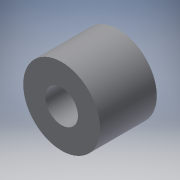
# Autodesk Inventor part: Espaçadores
Saved by Autodesk Inventor 2019 (Build 230136000, 136)
## iProperties
Created: 2020-05-30
Part Number: Espaçadores
Material: Generic
Document SubType Name: Modeling
Designer: luiza
Density: 1 g/cm^3
Appearance: Default
Author: luiza
Autodesk Inventor part; units mm, degrees
ref_plane "YZ Plane" through (0, 0, 0) normal (1, 0, 0) x (0, 1, 0)
ref_plane "Work Plane1" through (0, 0, 9.3133) normal (0, 0, 1) x (1, 0, 0)
sketch "Sketch1" plane through (0, 0, 9.3133) normal (0, 0, 1) x (1, 0, 0)
  circle A0 centre (44, 32.5) radius 1.5 projected
  circle A1 centre (44, 32.5) radius 4
  circle A2 centre (44, 32.5) radius 1.7
  point P0 (0, 0)
  dimension "d0" = 2.5
  dimension "d1" = 0.2
  constraints: 2 centre point
  measures "d0" radial gap between concentric circles of A0 A1
  measures "d1" radial gap between concentric circles of A0 A2
ref_plane "Work Plane2" through (41.5, 30, 4.899) normal (0, 0, -1) x (0, 1, 0)
extrude "Extrusion1" add sketch "Sketch1" against normal blind 5.9 contours A1
body "Solid1"
